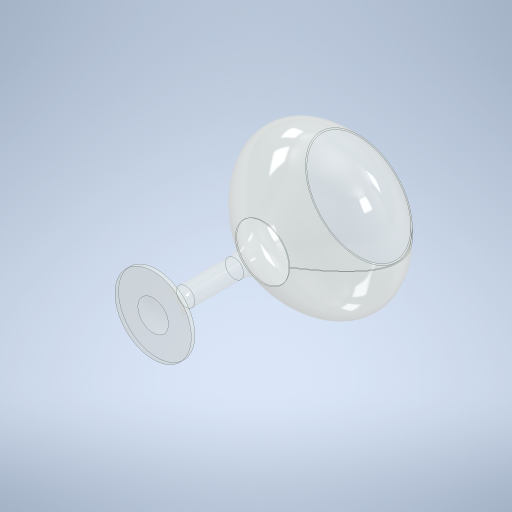
# Autodesk Inventor part: Glas
Saved by Autodesk Inventor 2024 (Build 280153000, 153)
## iProperties
Created: 2024-03-21
Part Number: Glas
Material: Glas
Document SubType Name: Modeling
Designer: ffogue
Density: 2.18 g/cm^3
Appearance: Klar
Author: ffogue
Autodesk Inventor part; units mm, degrees
ref_plane "YZ Plane" through (0, 0, 0) normal (1, 0, 0) x (0, 1, 0)
ref_plane "XZ Plane" through (0, 0, 0) normal (0, 1, 0) x (-1, 0, 0)
sketch "Skizze1" plane through (0, 0, 0) normal (0, 0, 1) x (1, 0, 0)
  line L0 (0, 0) -> (0, 95)
  line L1 (0, 95) -> (52.5, 95)
  line L2 (52.5, 95) -> (70, 78.185) construction
  line L3 (70, 78.185) -> (100, 54.4042) construction
  line L4 (100, 54.4042) -> (60, 22.4311) construction
  line L5 (60, 22.4311) -> (26.3149, 0) construction
  spline S0 degree 4 poles (52.5, 95) (70, 78.185) (100, 54.4042) (60, 22.4311) (26.3149, 0) knots 1 1 1 1 1 2 2 2 2 2
  line L6 (0, 0) -> (26.3149, 0)
  dimension "d0" = 95
  dimension "d12" = 105
  dimension "d13" = 200
  dimension "d14" = 140
  dimension "d15" = 120
  dimension "d16" = 16.815
  dimension "d17" = 40.5958
  dimension "d18" = 72.5689
  dimension "d20" = 52.6298
  constraints: 6 end point, 1 horizontal, 1 horizontal alignment, 1 vertical, 3 other
  measures "d0" distance of L0.start L0.end
  measures "d12" diameter of L1.end L0
  measures "d13" diameter of L3.end L0
  measures "d14" diameter of L2.end L0
  measures "d15" diameter of L4.end L0
  measures "d16" vertical distance of L0.end L2.end
  measures "d17" vertical distance of L0.end L3.end
  measures "d18" vertical distance of L0.end L4.end
  measures "d20" diameter of L5.end L0
revolve "Umdrehung1" add sketch "Skizze1" angle 360 about axis through (0, 0, 0) along (0, 1, 0)
shell "Wandung1" thickness 1 removed faces 1 at (15.8747, 95, 30.7926)
ref_plane "Arbeitsebene1" through (0, 0, 0) normal (0, 0, 1) x (1, 0, 0)
sketch "Skizze3" plane through (0, 0, 0) normal (0, 0, 1) x (1, 0, 0)
  line L0 (26.3149, 0) -> (-26.3149, 0) projected
  line L1 (52.5, 95) -> (-52.5, 95) projected
  line L2 (51.0567, 95) -> (-51.0567, 95) projected
  line L3 (26.0122, 1) -> (-26.0122, 1) projected
  arc A0 (-9, -27.1862) -> (-26.3149, 0) centre (-39, -27.1862) ccw
  line L4 (0, 0) -> (0, -105)
  line L5 (-9, -27.1862) -> (-9, -75.1862)
  arc A1 (0, -103.1862) -> (-14.9609, -107.1862) centre (0, -133.1648) ccw
  line L6 (-14.9609, -107.1862) -> (-37.5, -107.1862)
  line L7 (-37.5, -107.1862) -> (-37.5, -103.6862)
  arc A2 (-37.5, -103.6862) -> (-9, -75.1862) centre (-37.5, -75.1862) ccw
  point P0 (-37.5, -105.4362)
  point P1 (0, -52.5)
  dimension "d24" = 200
  dimension "d25" = 30
  dimension "d26" = 80
  dimension "d27" = 75
  dimension "d28" = 4
  dimension "d30" = 9
  dimension "d32" = 29.9218
  dimension "d33" = 3.5
  constraints: 8 end point, 6 point on circle, 3 centre point, 3 midpoint, 2 point on line, 2 tangent, 2 vertical, 1 horizontal, 1 perpendicular, 1 vertical alignment, 2 other
  measures "d24" distance from line of L4.end L1
  measures "d25" radius of A0
  measures "d26" vertical distance of L6.end L5.start
  measures "d27" diameter of point (-37.5, -105.436) L4
  measures "d28" vertical distance of L6.start A1.start
  measures "d30" distance from line of L5 point (0, -52.5)
  measures "d32" diameter of L6.start L4
  measures "d33" distance of L6.end L7.end
revolve "Umdrehung2" add sketch "Skizze3" angle 360 about axis through (0, 0, 0) along (0, -1, 0)
